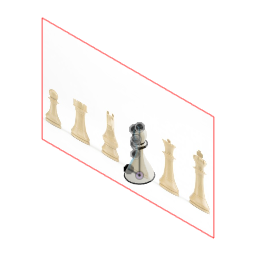
Bishop v3 (Autodesk Fusion 360 design; units mm, degrees)
Autodesk Fusion 360 part; units mm, degrees
sketch "Sketch1" plane through (0, 0, 0) normal (0, 1, 0) x (1, 0, 0)
  line L0 (0, 0) -> (0, -80)
  line L1 (0, 0) -> (-20, 0)
  line L2 (-6.0501, -55.2545) -> (-10.2637, -52.2049)
  line L3 (-10.4525, -50.8951) -> (-5.4129, -45.8555)
  line L4 (-10.2637, -52.2049) -> (-10.4525, -50.8951)
  line L5 (0, -70.5202) -> (-2.9993, -80)
  line L6 (-2.9993, -80) -> (0, -80)
  spline S0 degree 5 poles (-20, 0) (-20, -0.6734) (-19.8627, -2.1332) (-19.2448, -4.6616) (-17.6673, -8.6584) (-14.8349, -14.4044) (-11.653, -20.5245) (-8.6578, -26.6258) (-6.3321, -32.3545) (-5.0054, -37.4666) (-4.7896, -41.8717) (-5.5103, -44.8202) (-6.5359, -46.7178) (-7.4317, -47.8457) (-7.9327, -48.3753) knots 0 0 0 0 0 0 0.1 0.2 0.3 0.4 0.5 0.6 0.7 0.8 0.9 1 1 1 1 1 1
  spline S1 degree 5 poles (-6.6133, -54.8469) (-6.9485, -55.5323) (-7.579, -56.8841) (-8.4052, -58.855) (-9.2635, -61.3672) (-9.9029, -64.3011) (-10.0667, -67.0089) (-9.7113, -69.4697) (-8.8041, -71.6681) (-7.3543, -73.6084) (-5.3976, -75.3076) (-3.4574, -76.4886) (-1.8044, -77.2803) (-0.6159, -77.767) (0, -78) knots 0 0 0 0 0 0 0.1 0.2 0.3 0.4 0.5 0.6 0.7 0.8 0.9 1 1 1 1 1 1
  line L7 (-20, 3) -> (-20, -3)
  point P0 (-7, -31)
  point P1 (-9.3943, -69.9909)
  dimension "d2" = 20
  dimension "d5" = 80
  dimension "d7" = 45
  constraint coincident L0.start L1.start
  constraint vertical L0
  constraint perpendicular L0 L1
  constraint coincident L0 L5.start
  constraint perpendicular L0 L6
  constraint coincident L0.end L6.end
  constraint coincident L3 S0.end
  constraint midpoint L3 S0.end
  constraint coincident L2 S1.start
  constraint coincident L0 S1.end
  constraint midpoint L1.end L7
  measures "d2" distance of L0.start L1.end
  measures "d5" distance of L0.start L0.end
  measures "d7" angle of L0 L3
revolve "Revolve1" add sketch "Sketch1" angle 360 about axis through (0, 0, 0) along (0, 0, 1)
sketch "Sketch2" plane through (0, 0, 0) normal (0, 1, 0) x (1, 0, 0)
  line L0 (-5.5, -78) -> (-0.7405, -62.5113)
  line L1 (-0.7405, -62.5113) -> (1.027, -63.0544)
  line L2 (1.027, -63.0544) -> (-3.8706, -78.9928)
  arc A0 (1.027, -63.0544) -> (-0.7405, -62.5113) centre (0.1432, -62.7828) ccw
  line L3 (-5.5, -78) -> (-3.8706, -78.9928)
  constraint perpendicular L0 L1
  constraint perpendicular L1 L2
extrude "Extrude1" cut sketch "Sketch2" along normal through all and the other way through all
equation "d1 = 8 cm"
equation "d2 = d1 * 1 / 4"
